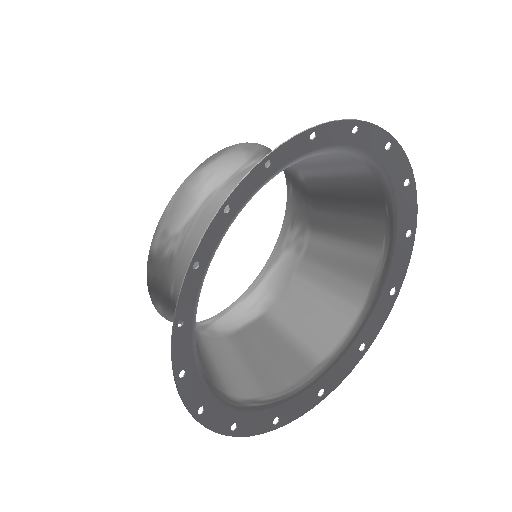
# Autodesk Inventor part: inlet cone
Saved by Autodesk Inventor 2022 (Build 260148000, 148)
## iProperties
Created: 2007-05-11
Part Number: inlet cone
Document SubType Name: Modeling
Designer: LionelF
Material: Steel, Mild
Density: 7.86 g/cm^3
Mass: 9657.51 g
Surface Area: 10436.6 cm^2
Volume: 1228.69 cm^3
Appearance: Steel
Autodesk Inventor part; units mm, degrees
ref_plane "YZ Plane" through (0, 0, 0) normal (1, 0, 0) x (0, 1, 0)
ref_plane "XZ Plane" through (0, 0, 0) normal (0, 1, 0) x (-1, 0, 0)
ref_plane "XY Plane" through (0, 0, 0) normal (0, 0, 1) x (1, 0, 0)
sketch "Sketch1" plane through (0, 0, 0) normal (0, 0, 1) x (1, 0, 0)
  line L0 (3092.83, 432.2356) -> (3090.4487, 432.2356)
  line L1 (2947.7667, 269.7223) -> (3077.9198, 348.6127)
  line L2 (2946.5323, 271.7587) -> (3076.6855, 350.6491)
  arc A0 (3077.9198, 348.6127) -> (3092.83, 375.0856) centre (3061.8737, 375.0856) ccw
  arc A1 (3076.6855, 350.6491) -> (3090.4487, 375.0856) centre (3061.8737, 375.0856) ccw
  arc A2 (2863.2209, 274.0445) -> (2947.7667, 269.7223) centre (2908.68, 334.2074) ccw
  arc A3 (2863.2209, 277.0574) -> (2946.5323, 271.7587) centre (2908.68, 334.2074) ccw
  line L3 (2863.2209, 67.1106) -> (3092.83, 67.1106) construction
  line L4 (3090.4487, 375.0856) -> (3090.4487, 432.2356)
  line L5 (2863.2209, 277.0574) -> (2863.2209, 274.0445)
  line L6 (3092.83, 432.2356) -> (3092.83, 375.0856)
  dimension "d0" = 30.9563
  dimension "d1" = 75.4062
  dimension "d2" = 30.9563
  dimension "d3" = 153.1937
  dimension "d4" = 229.6091
  dimension "d5" = 365.125
  dimension "d6" = 209.9469
  dimension "d7" = 307.975
  dimension "d8" = 267.0969
  dimension "d9" = 2.3813
  constraints: 14 end point, 8 point on circle, 5 tangent, 4 centre point, 1 concentric, 1 perpendicular
  measures "d0" radius of A0
  measures "d1" radius of A2
  measures "d2" distance from line of L6 A0.centre
  measures "d3" horizontal distance of A2.centre A0.centre
  measures "d4" distance from line of L5.start L6
  measures "d5" distance between parallel lines of L0 L3
  measures "d6" distance from line of L3 L5.start
  measures "d7" distance from line of L3 A0.centre
  measures "d8" distance from line of L3 A2.centre
  measures "d9" distance between parallel lines of L4 L6
revolve "Revolution1" add sketch "Sketch1" angle 360 about axis through (2863.2209, 67.1106, 0) along (1, 0, 0)
sketch "Sketch2" plane through (3092.83, 67.1106, 0) normal (1, 0, 0) x (0, 0, -1)
  circle A0 centre (0, 0) radius 307.975 projected
  circle A1 centre (0, 0) radius 365.125 projected
  point P0 (333.6081, 79.2847)
  dimension "d11" = 342.9
  dimension "d12" = 79.2847
  measures "d11" distance of A1.centre point (333.608, 79.285)
  measures "d12" vertical distance of A0.centre point (333.608, 79.285)
hole "Hole1" at (3092.83, 146.3953, -333.6081) direction (-1, 0, 0) diameter 19.05 end through all
pattern_circular "Circular Pattern1" count 16 over 360 about axis through (3091.6393, 67.1106, 0) along (1, 0, 0) of "Hole1"
body "Solid1"
